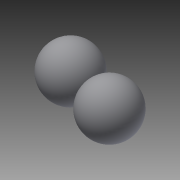
# Autodesk Inventor part: Cherry_fruit
Saved by Autodesk Inventor 2015 (Build 190159000, 159)
## iProperties
Created: 2015-04-11
Part Number: Cherry_fruit
Material: Generic
Document SubType Name: Modeling
Designer: tquinn
Density: 1 g/cm^3
Appearance: Default
Author: tquinn
Autodesk Inventor part; units mm, degrees
ref_plane "YZ Plane" through (0, 0, 0) normal (1, 0, 0) x (0, 1, 0)
ref_plane "XZ Plane" through (0, 0, 0) normal (0, 1, 0) x (-1, 0, 0)
sketch "Sketch1" plane through (0, 0, 0) normal (0, 0, 1) x (1, 0, 0)
  circle A0 centre (0, 0) radius 5.08
  line L0 (0, 5.08) -> (0, -5.08)
  dimension "d0" = 10.16
  constraints: 2 end point, 2 point on circle, 1 centre point, 1 coincident, 1 vertical
  measures "d0" diameter of A0
revolve "Revolution1" add sketch "Sketch1" angle 360 about axis through (0, 5.08, 0) along (0, -1, 0) picked at (-0.7869, -1.4994) contours L0 A0
ref_plane "Work Plane1" through (0, 0, -2.54) normal (0, 0, 1) x (1, 0, 0)
sketch "Sketch2" plane through (0, 0, -2.54) normal (0, 0, 1) x (1, 0, 0)
  circle A0 centre (-10.2575, 0) radius 5.08
  line L0 (-10.2575, 5.08) -> (-10.2575, -5.08)
  point P0 (0, 0)
  dimension "d3" = 10.16
  constraints: 2 end point, 2 point on circle, 1 centre point, 1 vertical
  measures "d3" diameter of A0
revolve "Revolution2" add sketch "Sketch2" angle 360 about axis through (-10.2575, 5.08, -2.54) along (0, -1, 0) picked at (-11.9385, 0.2041) contours L0 A0
body "Solid1"
